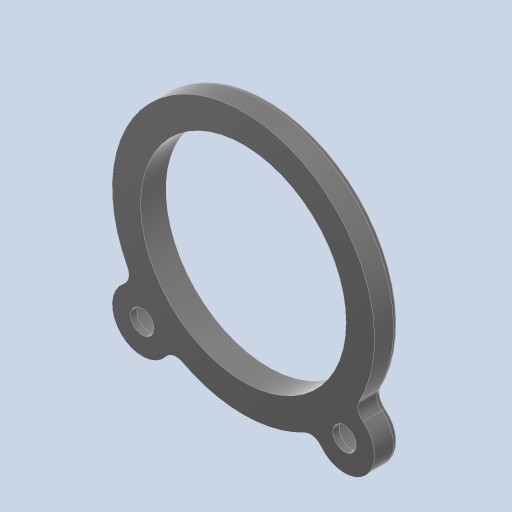
# Autodesk Inventor part: cage_inside_04
Saved by Autodesk Inventor 2024.4 (Build 284460030, 460C)
## iProperties
Created: 2026-05-04
Part Number: cage_inside_04
Material: PLA Plastic
Document SubType Name: Modeling
Designer: tooles01
Density: 1.06 g/cm^3
Appearance: Smooth - White(2)
Author: tooles01
Autodesk Inventor part; units mm, degrees
ref_plane "YZ Plane" through (0, 0, 0) normal (1, 0, 0) x (0, 1, 0)
ref_plane "XZ Plane" through (0, 0, 0) normal (0, 1, 0) x (-1, 0, 0)
ref_plane "XY Plane" through (0, 0, 0) normal (0, 0, 1) x (1, 0, 0)
derived "cage_outside_04.ipt"
sketch "Sketch1: base" plane through (0, 0, 0) normal (0, 0, 1) x (1, 0, 0)
  circle A0 centre (33, 30) radius 16.25
  line L0 (17, 46) -> (17, 14) construction
  line L1 (17, 14) -> (49, 14) construction
  circle A1 centre (33, 30) radius 17.75
  circle A2 centre (17, 14) radius 1.8 construction
  circle A3 centre (17, 14) radius 3.25 construction
  circle A4 centre (49, 14) radius 1.8 construction
  circle A5 centre (49, 14) radius 3.25 construction
  circle A6 centre (33, 30) radius 20.75
  circle A7 centre (17, 14) radius 4.75
  circle A8 centre (49, 14) radius 4.75
  point P0 (0, 0)
  point P1 (17, 30)
  point P2 (33, 14)
sketch "Sketch: base" plane through (0, 0, 0) normal (0, 0, 1) x (1, 0, 0)
  circle A0 centre (17, 14) radius 4.75 projected
  circle A1 centre (49, 14) radius 4.75 projected
  circle A2 centre (33, 30) radius 16.25 projected
  circle A3 centre (33, 30) radius 20.75 projected
  point P0 (0, 0)
  point P1 (50.3145, 18.5645)
  point P2 (15.6855, 18.5645)
  point P3 (21.5645, 12.6855)
  point P4 (44.4355, 12.6855)
extrude "Ex1: base" add sketch "Sketch: base" along normal blind 4
hole "Hole1" at (49, 14, 0) at (17, 14, 0) direction (0, 0, 1) diameter 3.7 end through all counterbore diameter 6.5 counterbore depth 3 clearance for "Socket Head Cap Screw" size "M3" standard "Ansi Metric M Profile"
fillet "Fillet2" radius 2 4 edges at (15.6855, 18.5645, 2) (21.5645, 12.6855, 2) (44.4355, 12.6855, 2) (50.3145, 18.5645, 2)
fillet "Fillet1" radius 1 1 edges at (33, 50.75, 0)
sketch "Sketch: text" plane through (0, 0, 0) normal (0, 0, -1) x (-1, 0, 0)
  line L0 (-34.75, 50) -> (-31.25, 50) construction
  line L1 (-31.25, 50) -> (-31.25, 46.5) construction
  line L2 (-31.25, 46.5) -> (-34.75, 46.5) construction
  line L3 (-34.75, 46.5) -> (-34.75, 50) construction
  line L4 (-35.8252, 48.935) -> (-34.9099, 48.935)
  line L5 (-34.9099, 48.935) -> (-34.4614, 47.4796)
  line L6 (-34.4614, 47.4796) -> (-34.0007, 48.935)
  line L7 (-34.0007, 48.935) -> (-33.1129, 48.935)
  line L8 (-33.1129, 48.935) -> (-34.0892, 46.6375)
  line L9 (-34.0892, 46.6375) -> (-34.8703, 46.6375)
  line L10 (-34.8703, 46.6375) -> (-35.8252, 48.935)
  line L11 (-31.4287, 47.2294) -> (-33.0336, 47.2294)
  line L12 (-33.0336, 47.2294) -> (-33.0336, 47.9556)
  line L13 (-33.0336, 47.9556) -> (-31.4287, 49.8625)
  line L14 (-31.4287, 49.8625) -> (-30.6599, 49.8625)
  line L15 (-30.6599, 49.8625) -> (-30.6599, 47.9129)
  line L16 (-30.6599, 47.9129) -> (-30.2632, 47.9129)
  line L17 (-30.2632, 47.9129) -> (-30.2632, 47.2294)
  line L18 (-30.2632, 47.2294) -> (-30.6599, 47.2294)
  line L19 (-30.6599, 47.2294) -> (-30.6599, 46.6375)
  line L20 (-30.6599, 46.6375) -> (-31.4287, 46.6375)
  line L21 (-31.4287, 46.6375) -> (-31.4287, 47.2294)
  line L22 (-31.4287, 47.9129) -> (-31.4287, 48.9136)
  line L23 (-31.4287, 48.9136) -> (-32.2769, 47.9129)
  line L24 (-32.2769, 47.9129) -> (-31.4287, 47.9129)
  point P0 (0, 0)
  point P1 (-33, 30)
  point P2 (-33, 46.5)
  dimension "d11" = 3.5
  dimension "d16" = 16.5
  constraints: 1 horizontal, 1 midpoint, 1 perpendicular, 1 vertical alignment, 2 other
  measures "d11" distance of L0.start L0.end
  measures "d16" distance from line of point (-33, 30) L2
extrude "Ex2: text" cut sketch "Sketch: text" against normal blind 1
body "Solid1"
